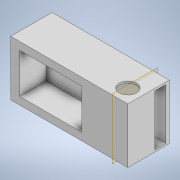
# Autodesk Inventor part: realcase
Saved by Autodesk Inventor 2022 (Build 260153000, 153)
## iProperties
Created: 2021-11-02
Part Number: realcase
Material: 일반
Document SubType Name: Modeling
Designer: ELEC-01
Density: 1 g/cm^3
Appearance: 기본값
Author: ELEC-01
Autodesk Inventor part; units mm, degrees
ref_plane "YZ Plane" through (0, 0, 0) normal (1, 0, 0) x (0, 1, 0)
ref_plane "XZ Plane" through (0, 0, 0) normal (0, 1, 0) x (-1, 0, 0)
ref_plane "XY Plane" through (0, 0, 0) normal (0, 0, 1) x (1, 0, 0)
sketch "스케치1" plane through (0, 0, 0) normal (0, 0, 1) x (1, 0, 0)
  line L0 (0, 0) -> (170, 0)
  line L1 (170, 0) -> (170, 80)
  line L2 (170, 80) -> (0, 80)
  line L3 (0, 80) -> (0, 0)
  dimension "d0" = 170
  dimension "d1" = 80
  constraints: 8 end point, 2 parallel, 1 horizontal, 1 perpendicular
  measures "d0" distance of L2.end L1.end
  measures "d1" distance of L1.end L0.end
extrude "돌출1" add sketch "스케치1" along normal mid plane 60
sketch "스케치3" plane through (0, 80, 30) normal (0, 1, 0) x (1, 0, 0)
  circle A0 centre (150, 20) radius 12.5
  line L0 (170, 0) -> (0, 0) projected
  line L1 (170, 60) -> (170, 0) projected
  point P0 (0, 30)
  dimension "d4" = 25
  dimension "d5" = 20
  dimension "d6" = 20
  constraints: 1 centre point
  measures "d4" diameter of A0
  measures "d5" distance from line of L0 A0.centre
  measures "d6" distance from line of L1 A0.centre
extrude "돌출2" cut sketch "스케치3" against normal blind 70
sketch "스케치4" plane through (170, 0, 30) normal (1, 0, 0) x (0, 0, -1)
  line L0 (39, 77) -> (55, 77)
  line L1 (55, 77) -> (55, 3)
  line L2 (55, 3) -> (39, 3)
  line L3 (39, 3) -> (39, 77)
  line L4 (60, 80) -> (0, 80) projected
  line L5 (60, 80) -> (60, 0) projected
  point P0 (30, 0)
  dimension "d9" = 16
  dimension "d10" = 74
  dimension "d11" = 3
  dimension "d12" = 5
  constraints: 8 end point, 2 parallel, 1 horizontal, 1 perpendicular
  measures "d9" distance of L1.end L2.end
  measures "d10" distance of L0.end L1.end
  measures "d11" distance between parallel lines of L4 L0
  measures "d12" distance between parallel lines of L5 L1
extrude "돌출3" cut sketch "스케치4" against normal blind 160
sketch "스케치5" plane through (0, 0, 30) normal (0, 0, 1) x (1, 0, 0)
  line L0 (13, 69) -> (103, 69)
  line L1 (103, 69) -> (103, 11)
  line L2 (103, 11) -> (13, 11)
  line L3 (13, 11) -> (13, 69)
  line L4 (170, 80) -> (0, 80) projected
  line L5 (0, 80) -> (0, 0) projected
  dimension "d15" = 90
  dimension "d16" = 58
  dimension "d17" = 11
  dimension "d18" = 13
  constraints: 8 end point, 2 parallel, 1 horizontal, 1 perpendicular
  measures "d15" distance of L1.end L2.end
  measures "d16" distance of L0.end L1.end
  measures "d17" distance between parallel lines of L4 L0
  measures "d18" distance between parallel lines of L3 L5
extrude "돌출4" cut sketch "스케치5" against normal blind 38.5
sketch "스케치9" plane through (13, 69, 30) normal (0, -1, 0) x (1, 0, 0)
  line L0 (90, 0) -> (90, -38.5) projected
  line L1 (90, -38.5) -> (70, -38.5)
  line L2 (70, -38.5) -> (70, -23.5)
  line L3 (70, -23.5) -> (90, -23.5)
  line L4 (90, -23.5) -> (90, -38.5)
  point P0 (-13, -30)
  dimension "d23" = 20
  dimension "d24" = 15
  constraints: 8 end point, 2 parallel, 1 horizontal, 1 perpendicular
  measures "d23" distance of L2.end L3.end
  measures "d24" distance of L1.end L2.end
extrude "돌출5" cut sketch "스케치9" against normal blind 8
sketch "스케치10" plane through (0, 0, -8.5) normal (0, 0, 1) x (1, 0, 0)
  line L0 (13, 69) -> (83, 69) projected
  line L1 (103, 77) -> (103, 11) projected
  line L2 (83, 69) -> (103, 69)
  line L3 (103, 69) -> (103, 77)
  line L4 (103, 77) -> (83, 77)
  line L5 (83, 77) -> (83, 69)
  point P0 (0, 0)
  constraints: 8 end point, 2 parallel, 1 horizontal, 1 perpendicular
extrude "돌출6" cut sketch "스케치10" against normal blind 1
sketch "스케치11" plane through (103, 11, 30) normal (-1, 0, 0) x (0, 0, 1)
  line L0 (-23.5, 58) -> (-23.5, 66)
  line L1 (-39, 46) -> (-39, 66)
  line L2 (-23.5, 66) -> (-39, 66)
  line L3 (-39, 66) -> (-39, 46)
  line L4 (-39, 46) -> (-23.5, 46)
  line L5 (-23.5, 46) -> (-23.5, 66)
  line L6 (-23.5, 66) -> (-39, 66) projected
  point P0 (-30, -11)
  point P1 (-39, 66)
  point P2 (-23.5, 66)
  point P3 (-39, 66)
  dimension "d31" = 20
  dimension "d32" = 0
  constraints: 12 end point, 1 horizontal, 1 parallel, 1 perpendicular
  measures "d31" distance between parallel lines of L4 L2
  measures "d32" distance between parallel lines of L6 L2
extrude "돌출7" cut sketch "스케치11" against normal blind 57
sketch "스케치13" plane through (170, 3, -9) normal (0, 0, -1) x (-1, 0, 0)
  line L0 (67, 66) -> (67, 8) projected
  line L1 (67, 66) -> (87, 66)
  line L2 (87, 66) -> (87, 54)
  line L3 (87, 54) -> (67, 54)
  line L4 (67, 54) -> (67, 66)
  line L5 (67, 54) -> (10, 54) projected
  line L6 (87, 74) -> (87, 66) projected
  point P0 (170, -3)
  point P1 (67, 54)
  dimension "d33" = 0
  dimension "d34" = 0
  constraints: 8 end point, 2 parallel, 1 horizontal, 1 perpendicular
  measures "d33" distance between parallel lines of L5 L3
  measures "d34" distance between parallel lines of L6 L2
extrude "돌출8" cut sketch "스케치13" against normal blind 2
ref_plane "작업 평면1" through (150, 0, 30) normal (1, 0, 0) x (0, 0, -1)
sketch "스케치14" plane through (150, 0, 30) normal (1, 0, 0) x (0, 0, -1)
  line L0 (42.5, 77) -> (2.5, 77)
  line L1 (2.5, 77) -> (2.5, 27)
  line L2 (2.5, 27) -> (42.5, 27)
  line L3 (42.5, 27) -> (42.5, 77)
  line L4 (0, 80) -> (0, 0) projected
  line L5 (7.5, 80) -> (32.5, 80) projected
  point P0 (30, 0)
  dimension "d38" = 40
  dimension "d39" = 2.5
  dimension "d40" = 3
  dimension "d41" = 50
  constraints: 8 end point, 2 parallel, 1 horizontal, 1 perpendicular
  measures "d38" distance of L0.start L0.end
  measures "d39" distance between parallel lines of L4 L1
  measures "d40" distance between parallel lines of L5 L0
  measures "d41" distance of L0.end L1.end
extrude "돌출9" cut sketch "스케치14" along normal blind 17 and the other way blind 71.125
